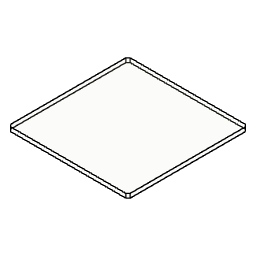
Polycarbonate Top v1 (Autodesk Fusion 360 design; units mm, degrees)
Autodesk Fusion 360 part; units mm, degrees
sketch "Sketch1" plane through (0, 0, 0) normal (0, 0, 1) x (1, 0, 0)
  line L0 (132.5, 137.5) -> (-132.5, 137.5)
  line L1 (-137.5, 132.5) -> (-137.5, -132.5)
  line L2 (-132.5, -137.5) -> (132.5, -137.5)
  line L3 (137.5, -132.5) -> (137.5, 132.5)
  line L4 (135, 135) -> (-137.5, -137.5) construction
  line L5 (-137.5, 137.5) -> (135, -135) construction
  line L6 (137.5, 132.5) -> (132.5, 137.5)
  line L7 (-137.5, -132.5) -> (-132.5, -137.5)
  line L8 (-132.5, 137.5) -> (-137.5, 132.5)
  line L9 (137.5, -132.5) -> (132.5, -137.5)
  dimension "d2" = 275
  dimension "d5" = 5
  dimension "d6" = 5
  dimension "d7" = 5
  dimension "d8" = 5
  dimension "d9" = 5
  dimension "d10" = 5
  constraint horizontal L0
  constraint perpendicular L0 L1
  constraint parallel L0 L2
  constraint parallel L1 L3
  constraint coincident L4 origin
  constraint coincident L5 origin
  constraint coincident L3.end L6.start
  constraint coincident L0.start L6.end
  constraint coincident L6 L4.start
  constraint coincident L1.end L7.start
  constraint coincident L2.start L7.end
  constraint perpendicular L4 L7
  constraint coincident L0.end L8.start
  constraint coincident L1.start L8.end
  constraint coincident L3.start L9.start
  constraint coincident L2.end L9.end
  constraint coincident L9 L5.end
  measures "d2" distance of L5.start L4.end
  measures "d5" distance of L2 L3.start
  measures "d6" distance of L3 L2.end
  measures "d7" distance of L1 L0.end
  measures "d8" distance of L0 L1.start
  measures "d9" distance of L2 L1.end
  measures "d10" distance of L1 L2.start
extrude "Extrude1" add sketch "Sketch1" along normal blind 9.525
equation "d11 = 3 / 8 * in"
